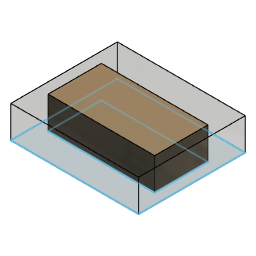
TCS34725_RGB Color Sensor v1 (Autodesk Fusion 360 design; units mm, degrees)
Autodesk Fusion 360 part; units mm, degrees
sketch "Sketch1" plane through (0, 0, 0) normal (0, 0, 1) x (1, 0, 0)
  line L0 (-1.2, 1) -> (1.2, 1)
  line L1 (1.2, 1) -> (1.2, -1)
  line L2 (1.2, -1) -> (-1.2, -1)
  line L3 (-1.2, -1) -> (-1.2, 1)
  line L4 (-1, 0.5) -> (1, 0.5)
  line L5 (1, 0.5) -> (1, -0.5)
  line L6 (1, -0.5) -> (-1, -0.5)
  line L7 (-1, -0.5) -> (-1, 0.5)
  constraint horizontal L0
  constraint vertical L1
  constraint horizontal L2
  constraint vertical L3
  constraint horizontal L4
  constraint vertical L5
  constraint horizontal L6
  constraint vertical L7
extrude "Extrude1" add sketch "Sketch1" along normal blind 0.6 makes body 1
extrude "Extrude2" add sketch "Sketch1" along normal blind 0.6 separate body contours L4 L5 L6 L7 makes body 2
